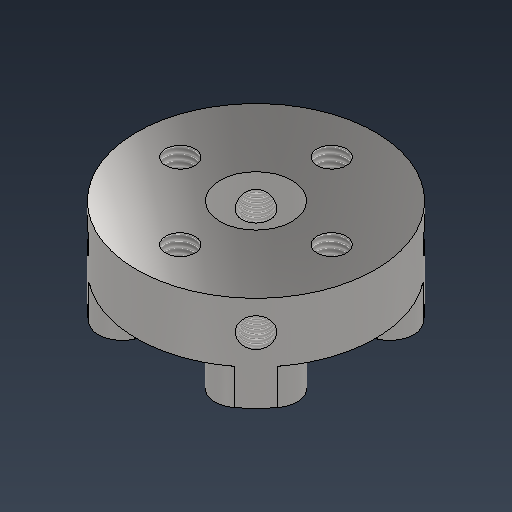
# Autodesk Inventor part: DiyHub
Saved by Autodesk Inventor 2026.2 (Build 302298010, 298A)
## iProperties
Created: 2026-04-20
Part Number: DiyHub
Material: Steel, Alloy
Document SubType Name: Modeling
Designer: szymo
Density: 7.73 g/cm^3
Appearance: Semi-Polished
Mass: 9.27765 g
Surface Area: 12.7709 cm^2
Volume: 1.20021 cm^3
Author: szymo
Autodesk Inventor part; units mm, degrees
ref_plane "XZ Plane" through (0, 0, 0) normal (0, 1, 0) x (-1, 0, 0)
sketch "Sketch1" plane through (0, 0, 0) normal (0, 1, 0) x (-1, 0, 0)
  circle A0 centre (0, 0) radius 15 construction
  circle A1 centre (0, 0) radius 10
  circle A2 centre (0, 0) radius 3
  circle A3 centre (0, 0) radius 6.35 construction
  circle A4 centre (6.35, 0) radius 3 construction
  line L0 (6.35, 0) -> (0, 0) construction
  circle A5 centre (6.35, 0) radius 2.5 construction
  circle A6 centre (0, 6.35) radius 2.5 construction
  circle A7 centre (0, 6.35) radius 3 construction
  circle A8 centre (-6.35, 0) radius 2.5 construction
  circle A9 centre (-6.35, 0) radius 3 construction
  circle A10 centre (0, -6.35) radius 2.5 construction
  circle A11 centre (0, -6.35) radius 3 construction
  circle A12 centre (0, 0) radius 5
  line L1 (-1.9685, -4.5962) -> (-3.937, -9.1924)
  line L2 (-4.5962, -1.9685) -> (-9.1924, -3.937)
  line L3 (-4.5962, 1.9685) -> (-9.1924, 3.937)
  line L4 (-1.9685, 4.5962) -> (-3.937, 9.1924)
  line L5 (3.937, 9.1924) -> (1.9685, 4.5962)
  line L6 (4.5962, 1.9685) -> (9.1924, 3.937)
  line L7 (4.5962, -1.9685) -> (9.1924, -3.937)
  line L8 (1.9685, -4.5962) -> (3.937, -9.1924)
  dimension "d2" = 20
  dimension "d4" = 12.7
  dimension "d77" = 10
  dimension "d0" = 30
  dimension "d1" = 5
  dimension "d3" = 6
  dimension "d5" = 6
  dimension "d6" = 5
  dimension "d9" = 360
  constraints: 18 end point, 10 centre point, 9 coincident, 8 tangent, 1 collinear, 1 horizontal, 1 horizontal alignment, 46 other
  measures "d0" diameter of A0
  measures "d3" diameter of A2
  measures "d5" diameter of A4
  measures "d6" diameter of A5
extrude "Extrusion1" add sketch "Sketch1" against normal blind 5
hole "Hole1" at (-6.35, 0, 0) at (0, 0, -6.35) at (6.35, 0, 0) at (0, 0, 6.35) direction (0, -1, 0) diameter 2.459 end through all thread size "M3x0.5" class "6H" standard "ISO Metric profile"
extrude "Extrusion2" add sketch "Sketch1" against normal blind 8 contours L6 A12 L5 A1 | A1 L8 A12 L7 | A12 | L4 A12 L3 A1 | A1 L2 A12 L1
fillet "Fillet1" radius 3 8 edges at (4.5962, -6.5, 1.9685) (4.5962, -6.5, -1.9685) (1.9685, -6.5, 4.5962) (-1.9685, -6.5, 4.5962) (-4.5962, -6.5, 1.9685) (-4.5962, -6.5, -1.9685) (-1.9685, -6.5, -4.5962) (1.9685, -6.5, -4.5962)
fillet "Fillet2" radius 2 8 edges at (3.937, -6.5, -9.1924) (9.1924, -6.5, -3.937) (9.1924, -6.5, 3.937) (3.937, -6.5, 9.1924) (-3.937, -6.5, 9.1924) (-9.1924, -6.5, 3.937) (-9.1924, -6.5, -3.937) (-3.937, -6.5, -9.1924)
ref_plane "Work Plane3" through (0, 0, 0) normal (-0.7071068, 0, 0.7071068) x (0, -1, 0)
ref_plane "Work Plane4" through (0, 0, 0) normal (0.7071068, 0, 0.7071068) x (0, 1, 0)
sketch "Sketch6" plane through (0, 0, 0) normal (-0.7071068, 0, 0.7071068) x (0, -1, 0)
  line L0 (5, -3) -> (0, -3) projected
  line L1 (5, 3) -> (0, 3) projected
  line L2 (5, -3) -> (0, 3)
  line L3 (5, 3) -> (0, -3)
  point P0 (0, 0)
  point P1 (2.5, 0)
  constraints: 4 end point, 1 midpoint
hole "Hole5" at (0, -2.5, 0) direction (0.7071068, 0, -0.7071068) diameter 2.459 depth 20 thread size "M3x0.5" class "6H" standard "ISO Metric profile"
hole "Hole6" at (0, -2.5, 0) direction (-0.7071068, 0, 0.7071068) diameter 2.459 depth 20 thread size "M3x0.5" class "6H" standard "ISO Metric profile"
sketch "Sketch7" plane through (0, 0, 0) normal (0.7071068, 0, 0.7071068) x (0, 1, 0)
  line L0 (-5, -3) -> (-5, 3) projected
  line L1 (0, 3) -> (0, -3) projected
  line L2 (-5, 3) -> (0, -3)
  line L3 (0, 3) -> (-5, -3)
  point P0 (0, 0)
  point P1 (-2.5, 0)
  constraints: 4 end point, 1 midpoint
hole "Hole7" at (0, -2.5, 0) direction (-0.7071068, 0, -0.7071068) diameter 2.459 depth 20 thread size "M3x0.5" class "6H" standard "ISO Metric profile"
hole "Hole8" at (0, -2.5, 0) direction (0.7071068, 0, 0.7071068) diameter 2.459 depth 20 thread size "M3x0.5" class "6H" standard "ISO Metric profile"
body "Solid1"
